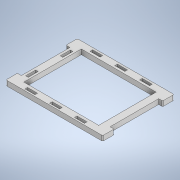
# Autodesk Inventor part: Bottom_bracket
Saved by Autodesk Inventor 2020 (Build 240168000, 168)
## iProperties
Created: 2019-06-20
Part Number: Bottom_bracket
Material: Generic
Document SubType Name: Modeling
Designer: Dammy
Density: 1 g/cm^3
Appearance: Default
Author: Dammy
Autodesk Inventor part; units mm, degrees
ref_plane "YZ Plane" through (0, 0, 0) normal (1, 0, 0) x (0, 1, 0)
ref_plane "XZ Plane" through (0, 0, 0) normal (0, 1, 0) x (-1, 0, 0)
ref_plane "XY Plane" through (0, 0, 0) normal (0, 0, 1) x (1, 0, 0)
sketch "Sketch1" plane through (0, 0, 0) normal (0, 1, 0) x (-1, 0, 0)
  line L0 (-89.5, 72) -> (89.5, 72)
  line L1 (89.5, 72) -> (89.5, -72)
  line L2 (89.5, -72) -> (-89.5, -72)
  line L3 (-89.5, -72) -> (-89.5, 72)
  line L4 (-89.5, 72) -> (89.5, -72) construction
  line L5 (89.5, 72) -> (-89.5, -72) construction
  line L6 (-75.5, 58) -> (75.5, 58)
  line L7 (75.5, 58) -> (75.5, -58)
  line L8 (75.5, -58) -> (-75.5, -58)
  line L9 (-75.5, -58) -> (-75.5, 58)
  line L10 (-75.5, 58) -> (75.5, -58) construction
  line L11 (75.5, 58) -> (-75.5, -58) construction
  line L12 (-89.5, -72) -> (-95.5, -72)
  line L13 (-97.5, -70) -> (-97.5, -51)
  line L14 (-95.5, -49) -> (-89.5, -49)
  line L15 (-89.5, -49) -> (-89.5, -72)
  line L16 (-89.5, 72) -> (-95.5, 72)
  line L17 (-97.5, 70) -> (-97.5, 51)
  line L18 (-95.5, 49) -> (-89.5, 49)
  line L19 (-89.5, 49) -> (-89.5, 72)
  line L20 (89.5, -72) -> (95.5, -72)
  line L21 (97.5, -70) -> (97.5, -51)
  line L22 (95.5, -49) -> (89.5, -49)
  line L23 (89.5, -49) -> (89.5, -72)
  line L24 (89.5, 72) -> (95.5, 72)
  line L25 (97.5, 70) -> (97.5, 51)
  line L26 (95.5, 49) -> (89.5, 49)
  line L27 (89.5, 49) -> (89.5, 72)
  line L28 (62.5, -67.85) -> (42.3, -67.85)
  line L29 (42.3, -67.85) -> (42.3, -62.65)
  line L30 (42.3, -62.65) -> (62.5, -62.65)
  line L31 (62.5, -62.65) -> (62.5, -67.85)
  line L32 (-7.7, -67.85) -> (-7.7, -62.65)
  line L33 (12.5, -62.65) -> (12.5, -67.85)
  line L34 (-7.7, -62.65) -> (12.5, -62.65)
  line L35 (12.5, -67.85) -> (-7.7, -67.85)
  line L36 (-57.7, -67.85) -> (-57.7, -62.65)
  line L37 (-37.5, -62.65) -> (-37.5, -67.85)
  line L38 (-57.7, -62.65) -> (-37.5, -62.65)
  line L39 (-37.5, -67.85) -> (-57.7, -67.85)
  line L40 (42.3, 63.65) -> (42.3, 68.85)
  line L41 (62.5, 68.85) -> (62.5, 63.65)
  line L42 (42.3, 68.85) -> (62.5, 68.85)
  line L43 (62.5, 63.65) -> (42.3, 63.65)
  line L44 (-7.7, 63.65) -> (-7.7, 68.85)
  line L45 (12.5, 68.85) -> (12.5, 63.65)
  line L46 (-7.7, 68.85) -> (12.5, 68.85)
  line L47 (12.5, 63.65) -> (-7.7, 63.65)
  line L48 (-57.7, 63.65) -> (-57.7, 68.85)
  line L49 (-37.5, 68.85) -> (-37.5, 63.65)
  line L50 (-57.7, 68.85) -> (-37.5, 68.85)
  line L51 (-37.5, 63.65) -> (-57.7, 63.65)
  arc A0 (95.5, -72) -> (97.5, -70) centre (95.5, -70) ccw
  arc A1 (97.5, -51) -> (95.5, -49) centre (95.5, -51) ccw
  arc A2 (95.5, 49) -> (97.5, 51) centre (95.5, 51) ccw
  arc A3 (97.5, 70) -> (95.5, 72) centre (95.5, 70) ccw
  arc A4 (-95.5, 72) -> (-97.5, 70) centre (-95.5, 70) ccw
  arc A5 (-97.5, 51) -> (-95.5, 49) centre (-95.5, 51) ccw
  arc A6 (-95.5, -49) -> (-97.5, -51) centre (-95.5, -51) ccw
  arc A7 (-97.5, -70) -> (-95.5, -72) centre (-95.5, -70) ccw
  line L52 (84.7, -45) -> (79.5, -45)
  line L53 (79.5, -45) -> (79.5, -24.8)
  line L54 (79.5, -24.8) -> (84.7, -24.8)
  line L55 (84.7, -24.8) -> (84.7, -45)
  line L56 (84.7, 45.2) -> (84.7, 25)
  line L57 (79.5, 25) -> (79.5, 45.2)
  line L58 (84.7, 25) -> (79.5, 25)
  line L59 (79.5, 45.2) -> (84.7, 45.2)
  point P0 (0, 0)
  point P1 (-97.5, -49)
  point P2 (-97.5, -72)
  point P3 (-97.5, 49)
  point P4 (-97.5, 72)
  point P5 (97.5, -49)
  point P6 (97.5, -72)
  point P7 (97.5, 49)
  point P8 (97.5, 72)
  dimension "d0" = 179
  dimension "d1" = 144
  dimension "d2" = 151
  dimension "d3" = 116
  dimension "d4" = 8
  dimension "d5" = 23
  dimension "d6" = 8
  dimension "d7" = 23
  dimension "d8" = 8
  dimension "d9" = 23
  dimension "d10" = 8
  dimension "d11" = 23
  dimension "d12" = 20.2
  dimension "d13" = 5.2
  dimension "d14" = 4.15
  dimension "d15" = 13
  dimension "d18" = 50
  dimension "d21" = 131.5
  dimension "d24" = 2
  dimension "d25" = 5.2
  dimension "d26" = 20.2
  dimension "d27" = 4
  dimension "d28" = 13
  dimension "d31" = 70
  constraints: 120 end point, 16 parallel, 16 point on circle, 16 point on line, 16 tangent, 9 horizontal, 8 centre point, 8 perpendicular, 7 equal radius, 4 midpoint, 2 vertical, 48 other
  measures "d0" distance of L1.end L2.end
  measures "d1" distance of L0.end L1.end
  measures "d2" distance of L7.end L8.end
  measures "d3" distance of L6.end L7.end
  measures "d4" distance of point (-97.5, -49) L14.end
  measures "d5" distance of point (-97.5, -72) point (-97.5, -49)
  measures "d6" distance of L18.end point (-97.5, 49)
  measures "d7" distance of point (-97.5, 49) point (-97.5, 72)
  measures "d8" distance of L22.end point (97.5, -49)
  measures "d9" distance of point (97.5, -49) point (97.5, -72)
  measures "d10" distance of point (97.5, 49) L26.end
  measures "d11" distance of point (97.5, 72) point (97.5, 49)
  measures "d12" distance of L29.end L30.end
  measures "d13" distance of L28.end L29.end
  measures "d14" distance between parallel lines of L2 L28
  measures "d15" distance between parallel lines of L7 L31
  measures "d18" distance of L28.end L32.start
  measures "d21" distance of L28.end L40.start
  measures "d24" radius of A0
  measures "d25" distance of L53.end L54.end
  measures "d26" distance of L52.end L53.end
  measures "d27" distance between parallel lines of L7 L53
  measures "d28" distance between parallel lines of L8 L52
  measures "d31" distance of L54.end L56.start
extrude "Extrusion1" add sketch "Sketch1" along normal blind 10
equation "\"d6\" = d4"
equation "\"d7\" = d5"
equation "\"d8\" = d4"
equation "\"d9\" = d5"
equation "\"d10\" = d4"
equation "\"d11\" = d5"
equation "\"d25\" = d13"
equation "\"d26\" = d12"
equation "\"d28\" = d15"
body "Solid1"
